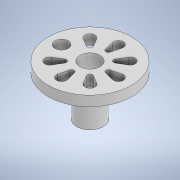
# Autodesk Inventor part: trục quay
Saved by Autodesk Inventor 2020 (Build 240168000, 168)
## iProperties
Created: 2022-11-23
Part Number: trục quay
Material: Generic
Document SubType Name: Modeling
Designer: ADMIN
Density: 1 g/cm^3
Appearance: Default
Author: ADMIN
Autodesk Inventor part; units mm, degrees
ref_plane "YZ Plane" through (0, 0, 0) normal (1, 0, 0) x (0, 1, 0)
ref_plane "XZ Plane" through (0, 0, 0) normal (0, 1, 0) x (-1, 0, 0)
ref_plane "XY Plane" through (0, 0, 0) normal (0, 0, 1) x (1, 0, 0)
sketch "Sketch1" plane through (0, 0, 0) normal (0, 1, 0) x (-1, 0, 0)
  circle A0 centre (0, 0) radius 4
  dimension "d0" = 8
  constraints: 1 centre point, 1 coincident
  measures "d0" diameter of A0
extrude "Extrusion1" add sketch "Sketch1" along normal blind 15
sketch "Sketch2" plane through (0, 15, 0) normal (0, 1, 0) x (1, 0, 0)
  circle A0 centre (0, 0) radius 3
  dimension "d3" = 6
  constraints: 1 centre point, 1 coincident
  measures "d3" diameter of A0
extrude "Extrusion2" cut sketch "Sketch2" against normal blind 13
sketch "Sketch3" plane through (0, 0, 0) normal (1, 0, 0) x (0, 1, 0)
  line L0 (15, -4) -> (15, 4) projected
  circle A0 centre (4, 0) radius 2
  line L1 (0, -4) -> (0, 4) projected
  point P0 (0, 0)
  dimension "d8" = 4
  dimension "d9" = 4
  constraints: 1 centre point
  measures "d8" diameter of A0
  measures "d9" distance from line of L1 A0.centre
extrude "Extrusion3" cut sketch "Sketch3" against normal blind 25
sketch "Sketch6" plane through (0, 15, 0) normal (0, 1, 0) x (1, 0, 0)
  circle A0 centre (0, 0) radius 12.5
  circle A1 centre (0, 0) radius 3 projected
  circle A2 centre (0, 0) radius 4
  dimension "d23" = 25
  constraints: 2 centre point, 2 coincident
  measures "d23" diameter of A0
extrude "Extrusion6" add sketch "Sketch6" against normal blind 3 contours A0
sketch "Sketch8" plane through (0, 15, 0) normal (0, 1, 0) x (1, 0, 0)
  circle A0 centre (-8.5, 0) radius 2
  circle A1 centre (0, 0) radius 12.5 projected
  arc A2 (8.1241, -1.4481) -> (8.1259, 1.4567) centre (8.5, 0.0041) ccw
  arc A3 (5.3129, 0.7322) -> (5.3121, -0.7202) centre (5.5, 0.0059) ccw
  line L0 (8.1259, 1.4567) -> (5.3129, 0.7322)
  line L1 (8.1241, -1.4481) -> (5.3121, -0.7202)
  line L2 (10, 0.0048) -> (4.75, 0.0048)
  line L3 (0, 0) -> (9.0336, 0) construction
  line L4 (0, 0) -> (7.8566, 0) construction
  arc A4 (1.4528, 8.1269) -> (-1.4519, 8.1231) centre (0, 8.5) ccw
  arc A5 (-0.7221, 5.3116) -> (0.7303, 5.3134) centre (0.0038, 5.5) ccw
  line L5 (1.4528, 8.1269) -> (0.7303, 5.3134)
  line L6 (-1.4519, 8.1231) -> (-0.7221, 5.3116)
  line L7 (0, 0) -> (7.2708, 0) construction
  arc A6 (6.7739, 4.7192) -> (4.7173, 6.7706) centre (6.0104, 6.0104) ccw
  arc A7 (3.2452, 4.2665) -> (4.2735, 3.2408) centre (3.8918, 3.8864) ccw
  line L8 (6.7739, 4.7192) -> (4.2735, 3.2408)
  line L9 (4.7173, 6.7706) -> (3.2452, 4.2665)
  arc A8 (-1.4567, -8.1259) -> (1.4481, -8.1241) centre (-0.0041, -8.5) ccw
  arc A9 (0.7202, -5.3121) -> (-0.7322, -5.3129) centre (-0.0059, -5.5) ccw
  line L10 (-1.4567, -8.1259) -> (-0.7322, -5.3129)
  line L11 (1.4481, -8.1241) -> (0.7202, -5.3121)
  line L12 (-0.0048, -10) -> (-0.0048, -4.75)
  arc A10 (-6.7706, -4.7173) -> (-4.7192, -6.7739) centre (-6.0104, -6.0104) ccw
  line L13 (-4.7192, -6.7739) -> (-3.2408, -4.2735)
  line L14 (-7.0267, -7.1137) -> (-3.3168, -3.4038)
  arc A11 (-3.2408, -4.2735) -> (-4.2665, -3.2452) centre (-3.8864, -3.8918) ccw
  line L15 (-6.7706, -4.7173) -> (-4.2665, -3.2452)
  arc A12 (-4.7269, 6.7706) -> (-6.7835, 4.7192) centre (-6.02, 6.0104) ccw
  line L16 (-6.7835, 4.7192) -> (-4.2831, 3.2408)
  arc A13 (-4.2831, 3.2408) -> (-3.2548, 4.2665) centre (-3.9014, 3.8864) ccw
  line L17 (-4.7269, 6.7706) -> (-3.2548, 4.2665)
  arc A14 (4.2569, -3.2452) -> (3.2312, -4.2735) centre (3.8768, -3.8918) ccw
  line L18 (4.7096, -6.7739) -> (3.2312, -4.2735)
  arc A15 (4.7096, -6.7739) -> (6.761, -4.7173) centre (6.0008, -6.0104) ccw
  line L19 (6.761, -4.7173) -> (4.2569, -3.2452)
  point P0 (6.3877, 6.3877)
  point P1 (5.5555, 5.5555)
  point P2 (5.1412, 5.1412)
  point P3 (0, -9.0336)
  point P4 (0, -7.8566)
  point P5 (0, -7.2708)
  point P6 (-6.3877, -6.3877)
  point P7 (-5.5555, -5.5555)
  point P8 (-5.1412, -5.1412)
  point P9 (-6.3973, 6.3877)
  point P10 (-5.5651, 5.5555)
  point P11 (-5.1508, 5.1412)
  dimension "d37" = 8.5
  dimension "d38" = 3
  dimension "d39" = 8.5
  dimension "d40" = 1.5
  dimension "d41" = 3
  constraints: 40 end point, 34 point on circle, 15 centre point, 15 symmetric about line, 4 horizontal, 4 tangent, 4 other
  measures "d37" distance of L3.start A0.centre
  measures "d38" diameter of A2
  measures "d39" distance of L3.start A2.centre
  measures "d40" diameter of A3
  measures "d41" distance of A2.centre A3.centre
extrude "Extrusion7" cut sketch "Sketch8" against normal blind 3 contours A0 | L1 A3 L2 A2 | L2 A3 L0 A2 | L5 A5 L6 A4 | L8 A7 L9 A6 | L10 A9 L12 A8 | L12 A9 L11 A8 | L15 A11 L14 A10 | L14 A11 L13 A10 | L17 A13 L16 A12 | L19 A15 L18 A14
body "Solid1"
